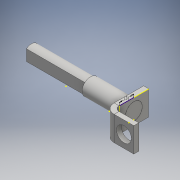
# Autodesk Inventor part: mocowanie_luzem
Saved by Autodesk Inventor 2016 (Build 200138000, 138)
## iProperties
Created: 2015-11-13
Part Number: mocowanie_luzem
Material: Ogólny
Document SubType Name: Sheet Metal
Designer: Mrianura
Density: 1 g/cm^3
Sheet Metal Rule: Domyślny_mm
Appearance: Domyślna
Author: Mrianura
Autodesk Inventor part; units mm, degrees
ref_plane "YZ Plane" through (0, 0, 0) normal (1, 0, 0) x (0, 1, 0)
ref_plane "XZ Plane" through (0, 0, 0) normal (0, 1, 0) x (-1, 0, 0)
ref_plane "XY Plane" through (0, 0, 0) normal (0, 0, 1) x (1, 0, 0)
sketch "Szkic1" plane through (0, 0, 0) normal (0, 1, 0) x (-1, 0, 0)
  line L0 (0, 0) -> (0, -5)
  line L1 (0, -5) -> (5, -5)
  line L2 (5, -5) -> (5, 0)
  line L3 (5, 0) -> (0, 0)
  line L4 (5, 0) -> (6, 0)
  line L5 (6, 0) -> (6, -1)
  line L6 (6, -1) -> (6, -5)
  line L7 (6, -5) -> (5, -5)
  dimension "d0" = 5
  dimension "d1" = 5
  dimension "d2" = 5
  dimension "d3" = 1
  dimension "d4" = 1
  dimension "d5" = 4
  measures "d0" distance of L0.start L0.end
  measures "d1" distance of L0.end L1.end
  measures "d2" distance of L1.end L2.end
  measures "d3" distance of L2.end L4.end
  measures "d4" distance of L4.end L5.end
  measures "d5" distance of L5.end L6.end
extrude "Płyta1" add sketch "Szkic1" along normal blind 1 contours L3 L2 L1 L0
sketch "Szkic2" plane through (-5, 0, 0) normal (0, 0, 1) x (1, 0, 0)
  point P0 (5, 0)
sketch "Szkic3" plane through (0, 1, 0) normal (0, 1, 0) x (1, 0, 0)
  point P0 (0, 0)
sketch "Szkic4" plane through (-4, 0, 0) normal (-1, 0, 0) x (0, -1, 0)
  line L0 (0, -5) -> (0, 0)
  line L1 (0, 0) -> (-8, 0)
  line L2 (-8, 0) -> (-8, -5)
  line L3 (-8, -5) -> (0, -5)
  constraints: 6 end point, 1 horizontal, 1 perpendicular, 1 vertical
edge flange "Kołnierz1" height 8 angle 90 thickness 1 bend radius 1 thickness toward (-1, 0, 0) relief straight relief width 1 relief depth 0.5 edges at (-5, 1, -2.5) wall of the first edge with corners at (-4, 0, -5) (-4, 0, 0) (-4, 8, 0) (-4, 8, -5)
bend "Gięcie1"
corner "Narożnik1"
sketch "Szkic5" plane through (-4, 8, 0) normal (1, 0, 0) x (0, 0, -1)
  line L0 (0, 0) -> (0, -6) projected
  line L1 (0, 0) -> (0, -3)
  line L2 (0, -3) -> (2.5, -3)
  circle A0 centre (2.5, -3) radius 1.725
  point P0 (0, -8)
  dimension "d17" = 3
  dimension "d18" = 2.5
  dimension "d19" = 3.45
  constraints: 4 end point, 1 centre point, 1 coincident, 1 midpoint, 1 perpendicular
  measures "d17" distance of L0.start L1.end
  measures "d18" distance of L1.end L2.end
  measures "d19" diameter of A0
sketch "Szkic6" plane through (-4, 8, 0) normal (1, 0, 0) x (0, 0, -1)
  line L0 (5, -6) -> (0, -6) projected
  line L1 (0, -6) -> (0, -3)
  line L2 (0, 0) -> (0, -6) projected
  point P0 (0, -8)
  dimension "d20" = 3
  constraints: 2 end point, 1 midpoint
  measures "d20" distance of L0.end L1.end
extrude "Wyciągnięcie proste1" cut sketch "Szkic5" against normal blind 10
sketch "Szkic7" plane through (-4, 8, 0) normal (1, 0, 0) x (0, 0, -1)
  point P0 (0, -8)
sketch "Szkic8" plane through (0, 1, 0) normal (0, 1, 0) x (1, 0, 0)
  line L0 (0, 0) -> (1, 0)
  line L1 (0, 0) -> (-3, 0)
  line L2 (1, 0) -> (1, 5)
  line L3 (0, 5) -> (0, 0)
  line L4 (1, 5) -> (0, 5)
  dimension "d23" = 1
  dimension "d24" = 5
  measures "d23" distance of L0.start L0.end
  measures "d24" distance of L0.end L2.end
sheet face with bend "Powierzchnia2" sketch "Szkic8" thickness 1 toward (0, -1, 0) bend radius 1 relief straight relief width 1 relief depth 0.5
bend "Gięcie2"
sketch "Szkic9" plane through (0, 1, 0) normal (0, 1, 0) x (1, 0, 0)
  line L0 (0, 0) -> (-1, 0)
  line L1 (1, 0) -> (-3, 0) projected
  line L2 (-1, 0) -> (-1, 2.5)
  circle A0 centre (-1, 2.5) radius 1.5
  dimension "d30" = 1
  dimension "d31" = 2.5
  dimension "d32" = 3
  constraints: 4 end point, 1 centre point, 1 coincident, 1 midpoint, 1 perpendicular
  measures "d30" distance of L0.start L0.end
  measures "d31" distance of L0.end L2.end
  measures "d32" diameter of A0
extrude "Wyciągnięcie proste2" cut sketch "Szkic9" against normal blind 10
sketch "Szkic10" plane through (-4, 8, 0) normal (1, 0, 0) x (0, 0, -1)
  line L0 (0, 0) -> (0, -6) projected
  line L1 (0, -3) -> (2.5, -3)
  circle A0 centre (2.5, -3) radius 1.7
  point P0 (0, -8)
  dimension "d35" = 2.5
  dimension "d36" = 3.4
  constraints: 2 end point, 1 centre point, 1 coincident, 1 horizontal, 1 midpoint
  measures "d35" distance of L1.start L1.end
  measures "d36" diameter of A0
extrude "Wyciągnięcie proste3" add sketch "Szkic10" against normal blind 8.8
sketch "Szkic11" plane through (-12.8, 5, -2.5) normal (-1, 0, 0) x (0, 0, 1)
  circle A0 centre (0, 0) radius 1.5
  line L0 (0, 1.5) -> (0, -1)
  line L1 (0, 1.5) -> (2.5, 1.5) construction
  line L2 (0, -1) -> (-1.118, -1)
  line L3 (0, -1) -> (1.118, -1)
  point P0 (2.5, -5)
  dimension "d39" = 3
  dimension "d40" = 2.5
  dimension "d41" = 90
  constraints: 8 end point, 3 point on circle, 2 perpendicular, 1 centre point, 1 horizontal, 1 point on line, 1 vertical
  measures "d39" diameter of A0
  measures "d40" distance of L0.start L0.end
  measures "d41" angle of L0 L1
sketch "Szkic12" plane through (-12.8, 5, -2.5) normal (-1, 0, 0) x (0, 0, 1)
  point P0 (2.5, -5)
extrude "Wyciągnięcie proste4" add sketch "Szkic11" along normal blind 12 contours A0 L3 L0 | L0 L2 A0
equation "\"d7\" = SzerokośćGięciaPodcięcia"
equation "\"d8\" = GłębokośćGięciaPodcięcia"
equation "\"d9\" = MinimalnaPozostałość"
equation "\"d10\" = PromieńGięcia"
equation "\"d13\" = PromieńGięcia"
equation "\"d14\" = RozmiarPodcięciaNarożnika"
equation "\"d15\" = Wielk_odstępu"
equation "\"d16\" = Rozmiar_promienia_Jacobiego"
equation "\"d25\" = PromieńGięcia"
equation "\"d26\" = SzerokośćGięciaPodcięcia"
equation "\"d28\" = MinimalnaPozostałość"
equation "\"d27\" = GłębokośćGięciaPodcięcia"
equation "\"d29\" = PromieńGięcia"
equation "\"PromieńGięcia\" = Grubość"
equation "\"SzerokośćGięciaPodcięcia\" = Grubość"
equation "\"GłębokośćGięciaPodcięcia\" = 0.5 * Grubość"
equation "\"RozmiarPodcięciaNarożnika\" = 4 * Grubość"
equation "\"MinimalnaPozostałość\" = 2 * Grubość"
equation "\"PromieńPrzejścia\" = PromieńGięcia"
equation "\"Rozmiar_promienia_Jacobiego\" = PromieńGięcia"
equation "\"Wielk_odstępu\" = Grubość"
equation "\"d6\" = PromieńGięcia"
equation "\"Grubość\" = 1"
